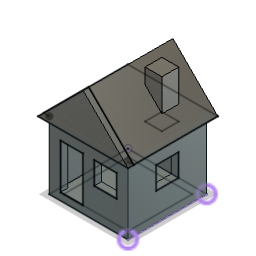
MMEZP_Domecek v1 (Autodesk Fusion 360 design; units mm, degrees)
Autodesk Fusion 360 part; units mm, degrees
sketch "Sketch1" plane through (0, 0, 0) normal (0, 1, 0) x (1, 0, 0)
  line L0 (0, 0) -> (35, 0)
  line L1 (35, 0) -> (35, -35)
  line L2 (35, -35) -> (0, -35)
  line L3 (0, -35) -> (0, 0)
  line L4 (3.2, -3.2) -> (31.8, -3.2)
  line L5 (31.8, -3.2) -> (31.8, -31.8)
  line L6 (31.8, -31.8) -> (3.2, -31.8)
  line L7 (3.2, -31.8) -> (3.2, -3.2)
  dimension "d1" = 35
  dimension "d2" = 35
  dimension "d4" = 3.2
  dimension "d5" = 3.2
  dimension "d6" = 3.2
  dimension "d7" = 3.2
  constraint horizontal L0
  constraint vertical L1
  constraint horizontal L2
  constraint vertical L3
  constraint coincident L0.start L3.end
  constraint horizontal L4
  constraint vertical L5
  constraint horizontal L6
  constraint vertical L7
  measures "d1" distance of L0.start L0.end
  measures "d2" distance of L0.end L1.end
  measures "d4" distance of L1 L5
  measures "d5" distance of L0 L4
  measures "d6" distance of L3 L7
  measures "d7" distance of L2 L6
extrude "Extrude1" add sketch "Sketch1" along normal blind 30 makes body 1
sketch "Sketch2" plane through (0, 0, 35) normal (0, 0, 1) x (1, 0, 0)
  line L0 (0, 0) -> (35, 0)
  line L1 (35, 0) -> (35, 30)
  line L2 (35, 30) -> (0, 30)
  line L3 (0, 30) -> (0, 0)
  line L4 (5, 23.2) -> (15, 23.2)
  line L5 (15, 23.2) -> (15, 3.2)
  line L6 (15, 3.2) -> (5, 3.2)
  line L7 (5, 3.2) -> (5, 23.2)
  line L8 (20, 13.2) -> (30, 13.2)
  line L9 (30, 13.2) -> (30, 23.2)
  line L10 (30, 23.2) -> (20, 23.2)
  line L11 (20, 23.2) -> (20, 13.2)
  line L12 (0, 30) -> (-2.5, 30)
  line L13 (35, 30) -> (37.5, 30)
  line L14 (-2.5, 30) -> (17.5, 50)
  line L15 (17.5, 50) -> (37.5, 30)
  dimension "d10" = 3.2
  dimension "d11" = 5
  dimension "d12" = 20
  dimension "d13" = 10
  dimension "d14" = 10
  dimension "d15" = 10
  dimension "d16" = 13.2
  dimension "d17" = 5
  dimension "d39" = 2.5
  dimension "d40" = 2.5
  dimension "d41" = 20
  dimension "d42" = 20
  constraint horizontal L4
  constraint vertical L5
  constraint horizontal L6
  constraint vertical L7
  constraint horizontal L8
  constraint vertical L9
  constraint horizontal L10
  constraint vertical L11
  constraint coincident L2.end L3.start
  constraint perpendicular L3 L12
  constraint coincident L1.end L2.start
  constraint perpendicular L1 L13
  measures "d10" distance of L0 L6
  measures "d11" distance of L3 L7
  measures "d12" distance of L4 L6
  measures "d13" distance of L5 L7
  measures "d14" distance of L9.end L10.end
  measures "d15" distance of L8.end L9.end
  measures "d16" distance of L0 L8
  measures "d17" distance of L1 L9
  measures "d39" distance of L2.end L12.end
  measures "d40" distance of L1.end L13.end
  measures "d41" distance of L2 L14.end
  measures "d42" horizontal distance of L13.end L14.end
extrude "Extrude2" add sketch "Sketch1" along normal blind 3.2 contours L4 L5 L6 L7 bodies 1
extrude "Extrude3" cut sketch "Sketch2" against normal blind 3.2 contours L4 L5 L6 L7 bodies 1
extrude "Extrude4" cut sketch "Sketch2" against normal blind 3.2 contours L8 L9 L10 L11 bodies 1
sketch "Sketch3" plane through (35, 0, 0) normal (1, 0, 0) x (0, 0, -1)
  line L0 (-35, 0) -> (0, 0)
  line L1 (0, 0) -> (0, 30)
  line L2 (0, 30) -> (-35, 30)
  line L3 (-35, 30) -> (-35, 0)
  line L4 (-22.5, 22.5) -> (-12.5, 22.5)
  line L5 (-12.5, 22.5) -> (-12.5, 12.5)
  line L6 (-12.5, 12.5) -> (-22.5, 12.5)
  line L7 (-22.5, 12.5) -> (-22.5, 22.5)
  line L8 (0, 0) -> (-35, 0)
  dimension "d24" = 10
  dimension "d25" = 10
  dimension "d26" = 12.5
  dimension "d27" = 12.5
  constraint horizontal L4
  constraint vertical L5
  constraint horizontal L6
  constraint vertical L7
  measures "d24" distance of L4.start L4.end
  measures "d25" distance of L4.start L6.end
  measures "d26" distance of L1 L5
  measures "d27" distance of L6 L8
extrude "Extrude5" cut sketch "Sketch3" against normal blind 35 contours L4 L5 L6 L7 bodies 1
sketch "Sketch4" plane through (0, 30, 0) normal (0, 1, 0) x (-1, 0, 0)
  line L0 (-31.8, 31.8) -> (-3.2, 31.8)
  line L1 (-3.2, 31.8) -> (-3.2, 3.2)
  line L2 (-3.2, 3.2) -> (-31.8, 3.2)
  line L3 (-31.8, 3.2) -> (-31.8, 31.8)
  line L4 (0, 35) -> (-35, 35)
  line L5 (-35, 35) -> (-35, 0)
  line L6 (-35, 0) -> (0, 0)
  line L7 (0, 0) -> (0, 35)
  line L8 (2.5, -2.5) -> (-37.5, -2.5)
  line L9 (-37.5, -2.5) -> (-37.5, 37.5)
  line L10 (-37.5, 37.5) -> (2.5, 37.5)
  line L11 (2.5, 37.5) -> (2.5, -2.5)
  line L12 (-30.8, 15.7) -> (-23.3, 15.7)
  line L13 (-23.3, 15.7) -> (-23.3, 8.2)
  line L14 (-23.3, 8.2) -> (-30.8, 8.2)
  line L15 (-30.8, 8.2) -> (-30.8, 15.7)
  dimension "d30" = 2.5
  dimension "d31" = 2.5
  dimension "d32" = 2.5
  dimension "d33" = 2.5
  dimension "d34" = 7.5
  dimension "d35" = 7.5
  dimension "d37" = 1
  dimension "d38" = 5
  constraint horizontal L8
  constraint vertical L9
  constraint horizontal L10
  constraint vertical L11
  constraint horizontal L12
  constraint vertical L13
  constraint horizontal L14
  constraint vertical L15
  measures "d30" distance of L7 L11
  measures "d31" distance of L5 L9
  measures "d32" distance of L6 L8
  measures "d33" distance of L4 L10
  measures "d34" distance of L13.end L14.end
  measures "d35" distance of L12.end L13.end
  measures "d37" distance of L3 L15
  measures "d38" distance of L2 L14
extrude "Extrude6" add sketch "Sketch2" along normal blind 2.5 separate body contours L2 L12 L13 L14 L15 makes body 2
extrude "Extrude7" add sketch "Sketch2" against normal blind 37.5 contours L2 L12 L13 L14 L15 bodies 1 2
extrude "Extrude8" add sketch "Sketch4" along normal blind 21 contours L12 L13 L14 L15 bodies 1
